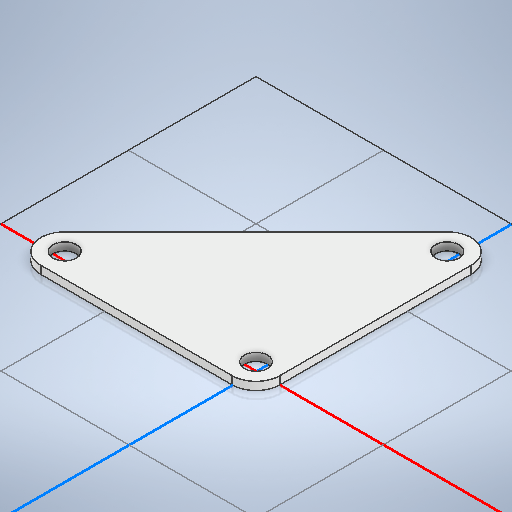
# Autodesk Inventor part: Triangle Gusset
Saved by Autodesk Inventor 2026 (Build 300175000, 175)
## iProperties
Created: 2025-04-06
Part Number: Triangle Gusset
Material: Acetal Resin, White
Document SubType Name: Modeling
Designer: avere
Density: 1.425 g/cm^3
Appearance: Smooth - White
Author: avere
Autodesk Inventor part; units mm, degrees
ref_plane "YZ Plane" through (0, 0, 0) normal (1, 0, 0) x (0, 1, 0)
ref_plane "XZ Plane" through (0, 0, 0) normal (0, 1, 0) x (-1, 0, 0)
ref_plane "XY Plane" through (0, 0, 0) normal (0, 0, 1) x (1, 0, 0)
sketch "Sketch1" plane through (0, 0, 0) normal (0, 1, 0) x (-1, 0, 0)
  circle A0 centre (0, 0) radius 2.3114
  circle A1 centre (38.1, 0) radius 2.3114
  circle A2 centre (0, -38.1) radius 2.3114
  arc A3 (0, 4.7625) -> (-4.7625, 0) centre (0, 0) ccw
  arc A4 (41.4676, -3.3676) -> (38.1, 4.7625) centre (38.1, 0) ccw
  arc A5 (-4.7625, -38.1) -> (3.3676, -41.4676) centre (0, -38.1) ccw
  line L0 (38.1, 4.7625) -> (0, 4.7625)
  line L1 (-4.7625, 0) -> (-4.7625, -38.1)
  line L2 (3.3676, -41.4676) -> (41.4676, -3.3676)
  dimension "d0" = 4.6228
  dimension "d1" = 4.6228
  dimension "d2" = 4.6228
  dimension "d3" = 9.525
  dimension "d4" = 9.525
  dimension "d5" = 9.525
  constraints: 6 centre point, 6 end point, 6 point on circle, 4 coincident, 4 tangent
  measures "d0" diameter of A0
  measures "d1" diameter of A1
  measures "d2" diameter of A2
  measures "d3" diameter of A3
  measures "d4" diameter of A4
  measures "d5" diameter of A5
extrude "Extrusion1" add sketch "Sketch1" along normal blind 1.5875
body "Solid1"
